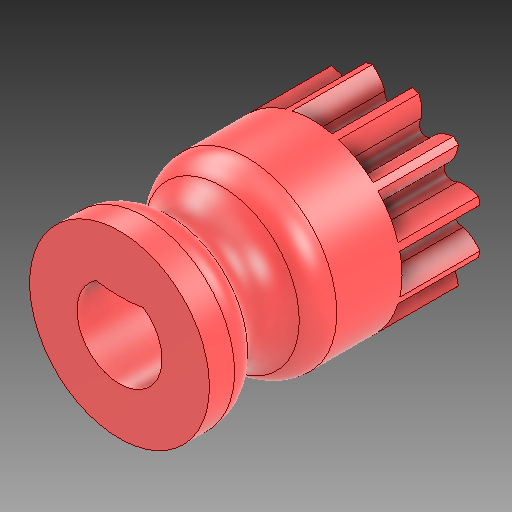
# Autodesk Inventor part: Drive Pinion 0.8m12t 2
Saved by Autodesk Inventor 2020.2 (Build 242310000, 310)
## iProperties
Created: 2020-03-17
Part Number: Drive Pinion 0.8m12t 2
Material: ABS Plastic
Document SubType Name: Modeling
Designer: Richard Hall
Density: 1.06 g/cm^3
Appearance: Satin -Light Red
Author: Richard Hall
Title: Exturder Pinion 0.8m12t
Autodesk Inventor part; units mm, degrees
ref_plane "YZ Plane" through (0, 0, 0) normal (1, 0, 0) x (0, 1, 0)
ref_plane "XZ Plane" through (0, 0, 0) normal (0, 1, 0) x (-1, 0, 0)
ref_plane "XY Plane" through (0, 0, 0) normal (0, 0, 1) x (1, 0, 0)
sketch "Sketch1" plane through (0, 0, 0) normal (0, 0, 1) x (1, 0, 0)
  spline S0 degree 3 poles (-1.2419, 5.4606) (-1.2, 5.4251) (-1.1163, 5.3542) (-0.998, 5.2397) (-0.8857, 5.1193) (-0.7811, 4.9922) (-0.7012, 4.8806) (-0.6427, 4.7878) (-0.6019, 4.7164) (-0.5644, 4.6431) (-0.5313, 4.5678) (-0.5022, 4.4907) (-0.4903, 4.4371) (-0.4844, 4.4103) knots 0 0 0 0 0.016452 0.032905 0.049357 0.065809 0.08226 0.090487 0.098713 0.10694 0.115166 0.123391 0.13161 0.13161 0.13161 0.13161
  spline S1 degree 3 poles (-0.4844, 4.4103) (-0.4816, 4.3741) (-0.4775, 4.3199) (-0.4661, 4.2482) (-0.4532, 4.1953) (-0.438, 4.143) (-0.4181, 4.0923) (-0.3949, 4.0431) (-0.3669, 3.9963) (-0.3344, 3.9525) (-0.2973, 3.9126) (-0.2557, 3.8773) (-0.2099, 3.8478) (-0.1606, 3.8244) (-0.1084, 3.8084) (-0.0545, 3.7999) (0, 3.8001) (0.0545, 3.7999) (0.1084, 3.8084) (0.1606, 3.8244) (0.2099, 3.8478) (0.2557, 3.8773) (0.2973, 3.9126) (0.3344, 3.9525) (0.3669, 3.9963) (0.3949, 4.0431) (0.4181, 4.0923) (0.438, 4.143) (0.4532, 4.1953) (0.4661, 4.2482) (0.4775, 4.3199) (0.4816, 4.3741) (0.4844, 4.4103) knots 0 0 0 0 0.010878 0.016318 0.021758 0.027199 0.032639 0.038079 0.043519 0.048959 0.054398 0.059836 0.065274 0.070713 0.076153 0.081591 0.087031 0.09247 0.097908 0.103348 0.108787 0.114225 0.119663 0.125102 0.130542 0.135983 0.141422 0.146862 0.152303 0.157744 0.163184 0.174061 0.174061 0.174061 0.174061
  spline S2 degree 3 poles (0.4844, 4.4103) (0.4903, 4.4371) (0.5022, 4.4907) (0.5313, 4.5678) (0.5644, 4.6431) (0.6019, 4.7164) (0.6427, 4.7878) (0.7012, 4.8806) (0.7811, 4.9922) (0.8857, 5.1193) (0.998, 5.2397) (1.1163, 5.3542) (1.2, 5.4251) (1.2419, 5.4606) knots 0 0 0 0 0.00822 0.016445 0.024671 0.032897 0.041124 0.04935 0.065801 0.082253 0.098705 0.115158 0.13161 0.13161 0.13161 0.13161
  circle A0 centre (0, 0) radius 3.8 construction
  circle A1 centre (0, 0) radius 4.4346 construction
  circle A2 centre (0, 0) radius 4.8 construction
  circle A3 centre (0, 0) radius 5.6
  point P0 (-1.1175, 5.3529)
  point P1 (-0.999, 5.2387)
  point P2 (-0.887, 5.1182)
  point P3 (-0.7826, 4.9911)
  point P4 (-0.6871, 4.8572)
  point P5 (-0.6432, 4.7875)
  point P6 (-0.6024, 4.7161)
  point P7 (-0.5651, 4.6428)
  point P8 (-0.532, 4.5675)
  point P9 (-0.5041, 4.4901)
  point P10 (-0.4741, 4.302)
  point P11 (-0.4653, 4.2483)
  point P12 (-0.4528, 4.1954)
  point P13 (-0.4372, 4.1433)
  point P14 (-0.4175, 4.0926)
  point P15 (-0.3941, 4.0435)
  point P16 (-0.3662, 3.9968)
  point P17 (-0.3336, 3.9532)
  point P18 (-0.2966, 3.9134)
  point P19 (-0.255, 3.8783)
  point P20 (-0.2093, 3.8488)
  point P21 (-0.1601, 3.8256)
  point P22 (-0.1081, 3.8096)
  point P23 (-0.0544, 3.8013)
  point P24 (0, 3.8)
  point P25 (0.0544, 3.8013)
  point P26 (0.1081, 3.8096)
  point P27 (0.1601, 3.8256)
  point P28 (0.2093, 3.8488)
  point P29 (0.255, 3.8783)
  point P30 (0.2966, 3.9134)
  point P31 (0.3336, 3.9532)
  point P32 (0.3662, 3.9968)
  point P33 (0.3941, 4.0435)
  point P34 (0.4175, 4.0926)
  point P35 (0.4372, 4.1433)
  point P36 (0.4528, 4.1954)
  point P37 (0.4653, 4.2483)
  point P38 (0.4741, 4.302)
  point P39 (0.5041, 4.4901)
  point P40 (0.532, 4.5675)
  point P41 (0.5651, 4.6428)
  point P42 (0.6024, 4.7161)
  point P43 (0.6432, 4.7875)
  point P44 (0.6871, 4.8572)
  point P45 (0.7826, 4.9911)
  point P46 (0.887, 5.1182)
  point P47 (0.999, 5.2387)
  point P48 (1.1175, 5.3529)
  constraints: 4 centre point, 2 point on circle, 113 other
extrude "Extrusion1" add sketch "Sketch1" against normal blind 5
extrude "Extrusion2" cut sketch "Sketch1" against normal blind 10 contours A3 S2 S1 S0 picked at (0.1377, 4.9372)
pattern_circular "Circular Pattern1" count 12 over 360 about axis through (0, 0, 0) along (0, 0, -1) of "Extrusion2"
sketch "Sketch2" plane through (0, 0, 0) normal (0, 0, 1) x (1, 0, 0)
  circle A0 centre (0, 0) radius 5.6
  arc A1 (1.6548, 5.3499) -> (1.2419, 5.4606) centre (0, 0) ccw projected
  constraints: 1 centre point, 1 coincident, 1 concentric
extrude "Extrusion3" add sketch "Sketch2" along normal blind 12
sketch "Sketch4" plane through (0, 0, 0) normal (1, 0, 0) x (0, 1, 0)
  circle A0 centre (6.1, 7.25) radius 2.05
  line L0 (5.6, 12) -> (-5.6, 12) projected
  line L1 (0, -8.003) -> (0, 13.0005) projected
  line L2 (5.3499, 0) -> (4.108, 0) projected
  point P0 (0, 0)
  point P1 (0, 12)
  dimension "d12" = 4.1
  dimension "d13" = 6.1
  dimension "d17" = 4.75
  constraints: 1 centre point, 1 midpoint
  measures "d12" diameter of A0
  measures "d13" horizontal distance of point (0, 12) A0.centre
  measures "d17" distance from line of A0.centre L0
revolve "Revolution1" cut sketch "Sketch4" angle 360 about axis through (0, 0, -10) along (0, 0, 1)
sketch "Sketch5" plane through (0, 0, 12) normal (0, 0, 1) x (1, 0, 0)
  arc A0 (-1.4808, 2.1977) -> (1.4808, 2.1977) centre (0, 0) ccw
  arc A1 (-1.4808, 2.1977) -> (1.4808, 2.1977) centre (0, 11.075) ccw
  arc A2 (1.4808, 2.1977) -> (-1.4808, 2.1977) centre (0, 0) ccw construction
  point P0 (0, 2.075)
  dimension "d18" = 5.3
  dimension "d19" = 9
  dimension "d20" = 2.075
  constraints: 7 point on circle, 3 centre point, 1 coincident, 1 horizontal alignment
  measures "d18" diameter of A0
  measures "d19" radius of A1
  measures "d20" distance of point (0, 0) point (0, 2.075)
extrude "Extrusion5" cut sketch "Sketch5" against normal through all
fillet "Fillet1" radius 2 4 edges at (3.9598, 3.9598, 5.2619) (-3.9598, -3.9598, 5.2619) (3.9598, 3.9598, 9.2381) (-3.9598, -3.9598, 9.2381)
equation "\"d0\" = FaceWidth"
equation "\"Module\" = 0.8"
equation "\"PressureAngle\" = 22.5deg"
equation "\"UnitProfileClearance\" = 0.25"
equation "\"UnitRoundRadius\" = 0.35"
equation "\"HeadDiameter\" = 11.2"
equation "\"RootDiameter\" = 7.6"
equation "\"BaseDiameter\" = 8.86924"
equation "\"PitchDiameter\" = 9.6"
equation "\"FaceWidth\" = 5"
equation "\"HelixAngle\" = 0"
equation "\"UnitCorrection\" = 0"
equation "\"UnitAddendumModification\" = 0"
equation "\"CircularPitch\" = 2.51327"
equation "\"UnitBacklashShift\" = 0"
equation "\"TotalToolShift\" = 0"
equation "\"IsInternal\" = 0"
body "Solid1"
